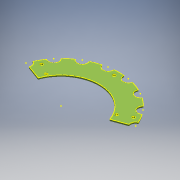
# Autodesk Inventor part: Board_Shape
Saved by Autodesk Inventor 2016 (Build 200138000, 138)
## iProperties
Created: 2015-07-29
Part Number: Board_Shape
Material: Generic
Document SubType Name: Modeling
Designer: bastli
Density: 1 g/cm^3
Appearance: Olive Green
Author: bastli
Autodesk Inventor part; units mm, degrees
ref_plane "YZ Plane" through (0, 0, 0) normal (1, 0, 0) x (0, 1, 0)
ref_plane "XZ Plane" through (0, 0, 0) normal (0, 1, 0) x (-1, 0, 0)
ref_plane "XY Plane" through (0, 0, 0) normal (0, 0, 1) x (1, 0, 0)
sketch "Sketch1" plane through (0, 0, 0) normal (0, 0, 1) x (1, 0, 0)
  arc A0 (65.342, -17.4038) -> (61.2418, -28.669) centre (63.542, -23.1274) ccw projected
  arc A1 (65.342, -17.4038) -> (65.342, 17.4038) centre (0, 0) ccw projected
  arc A2 (61.2418, 28.669) -> (65.342, 17.4038) centre (63.542, 23.1274) ccw projected
  arc A3 (61.2418, 28.669) -> (55.4489, 38.7025) centre (0, 0) ccw projected
  arc A4 (47.7431, 47.8859) -> (55.4489, 38.7025) centre (51.7999, 43.4653) ccw projected
  arc A5 (47.7431, 47.8859) -> (38.8679, 55.3331) centre (0, 0) ccw projected
  arc A6 (28.4859, 61.3272) -> (38.8679, 55.3331) centre (33.81, 58.5606) ccw projected
  arc A7 (28.4859, 61.3272) -> (17.5989, 65.2897) centre (0, 0) ccw projected
  arc A8 (5.7928, 67.3714) -> (17.5989, 65.2897) centre (11.7421, 66.5927) ccw projected
  arc A9 (5.7928, 67.3714) -> (-5.7928, 67.3714) centre (0, 0) ccw projected
  arc A10 (-17.5989, 65.2897) -> (-5.7928, 67.3714) centre (-11.7421, 66.5927) ccw projected
  arc A11 (-17.5989, 65.2897) -> (-28.4859, 61.3272) centre (0, 0) ccw projected
  arc A12 (-38.8679, 55.3331) -> (-28.4859, 61.3272) centre (-33.81, 58.5606) ccw projected
  arc A13 (-38.8679, 55.3331) -> (-47.7431, 47.8859) centre (0, 0) ccw projected
  arc A14 (-55.4489, 38.7025) -> (-47.7431, 47.8859) centre (-51.7999, 43.4653) ccw projected
  arc A15 (-55.4489, 38.7025) -> (-61.2418, 28.669) centre (0, 0) ccw projected
  arc A16 (-65.342, 17.4038) -> (-61.2418, 28.669) centre (-63.542, 23.1274) ccw projected
  arc A17 (-65.342, 17.4038) -> (-65.342, -17.4038) centre (0, 0) ccw projected
  arc A18 (-61.2418, -28.669) -> (-65.342, -17.4038) centre (-63.542, -23.1274) ccw projected
  arc A19 (-61.2418, -28.669) -> (-55.4489, -38.7025) centre (0, 0) ccw projected
  arc A20 (-47.7431, -47.8859) -> (-55.4489, -38.7025) centre (-51.7999, -43.4653) ccw projected
  arc A21 (-47.7431, -47.8859) -> (-38.8679, -55.3331) centre (0, 0) ccw projected
  arc A22 (-28.4859, -61.3272) -> (-38.8679, -55.3331) centre (-33.81, -58.5606) ccw projected
  arc A23 (-28.4859, -61.3272) -> (-17.5989, -65.2897) centre (0, 0) ccw projected
  arc A24 (-5.7928, -67.3714) -> (-17.5989, -65.2897) centre (-11.7421, -66.5927) ccw projected
  arc A25 (-5.7928, -67.3714) -> (5.7928, -67.3714) centre (0, 0) ccw projected
  arc A26 (17.5989, -65.2897) -> (5.7928, -67.3714) centre (11.7421, -66.5927) ccw projected
  arc A27 (17.5989, -65.2897) -> (28.4859, -61.3272) centre (0, 0) ccw projected
  arc A28 (38.8679, -55.3331) -> (28.4859, -61.3272) centre (33.81, -58.5606) ccw projected
  arc A29 (38.8679, -55.3331) -> (47.7431, -47.8859) centre (0, 0) ccw projected
  arc A30 (55.4489, -38.7025) -> (47.7431, -47.8859) centre (51.7999, -43.4653) ccw projected
  arc A31 (55.4489, -38.7025) -> (61.2418, -28.669) centre (0, 0) ccw projected
  circle A32 centre (0, 0) radius 44.3 projected
  circle A33 centre (-62.46, -8) radius 1.2 projected
  circle A34 centre (-46.46, 8) radius 1.2 projected
  circle A35 centre (62.46, -8) radius 1.2 projected
  circle A36 centre (46.46, 8) radius 1.2 projected
  circle A37 centre (62.46, 8) radius 1.2 projected
  circle A38 centre (46.46, -8) radius 1.2 projected
  circle A39 centre (-62.46, 8) radius 1.2 projected
  circle A40 centre (-46.46, -8) radius 1.2 projected
  circle A41 centre (-54.46, 0) radius 7.995 projected
  circle A42 centre (54.46, 0) radius 7.995 projected
  circle A43 centre (53.3645, -30.81) radius 1.55 projected
  circle A44 centre (39.6086, -47.2037) radius 1.55 projected
  circle A45 centre (16.1776, -44.4475) radius 1.55 projected
  circle A46 centre (0, -61.62) radius 1.55 projected
  circle A47 centre (-21.0753, -57.9039) radius 1.55 projected
  circle A48 centre (-30.4039, -36.2339) radius 1.55 projected
  circle A49 centre (-53.3645, -30.81) radius 1.55 projected
  circle A50 centre (53.3645, 30.81) radius 1.55 projected
  circle A51 centre (39.6086, 47.2037) radius 1.55 projected
  circle A52 centre (21.0753, 57.9039) radius 1.55 projected
  circle A53 centre (-40.963, 23.65) radius 1.55 projected
  circle A54 centre (-30.4039, 36.2339) radius 1.55 projected
  circle A55 centre (-16.1776, 44.4475) radius 1.55 projected
  circle A56 centre (0, 47.3) radius 1.55 projected
  circle A57 centre (0, 61.62) radius 1.55 projected
  circle A58 centre (-21.0753, 57.9039) radius 1.55 projected
  circle A59 centre (-39.6086, 47.2037) radius 1.55 projected
  circle A60 centre (-53.3645, 30.81) radius 1.55 projected
  circle A61 centre (16.1776, 44.4475) radius 1.55 projected
  circle A62 centre (30.4039, 36.2339) radius 1.55 projected
  circle A63 centre (40.963, 23.65) radius 1.55 projected
  circle A64 centre (-40.963, -23.65) radius 1.55 projected
  circle A65 centre (-39.6086, -47.2037) radius 1.55 projected
  circle A66 centre (-16.1776, -44.4475) radius 1.55 projected
  circle A67 centre (0, -47.3) radius 1.55 projected
  circle A68 centre (21.0753, -57.9039) radius 1.55 projected
  circle A69 centre (30.4039, -36.2339) radius 1.55 projected
  circle A70 centre (40.963, -23.65) radius 1.55 projected
  line L0 (-57.9039, 21.0753) -> (-41.6284, 15.1515)
  line L1 (41.6284, 15.1515) -> (57.9039, 21.0753)
  point P0 (0, 0)
  constraints: 4 end point, 4 point on circle, 2 line through centre
extrude "Extrusion1" add sketch "Sketch1" along normal blind 1.75 contours L1 A32 L0 A16 A15 A14 A13 A12 A11 A10 A9 A8 A7 A6 A5 A4 A3 A2
sketch "Sketch2" plane through (0, 0, 1.75) normal (0, 0, 1) x (1, 0, 0)
  circle A0 centre (-39.6086, 47.2037) radius 1.55 projected
  circle A1 centre (-30.4039, 36.2339) radius 1.55 projected
  circle A2 centre (-16.1776, 44.4475) radius 1.55 projected
  circle A3 centre (-21.0753, 57.9039) radius 1.55 projected
  circle A4 centre (16.1776, 44.4475) radius 1.55 projected
  circle A5 centre (21.0753, 57.9039) radius 1.55 projected
  circle A6 centre (30.4039, 36.2339) radius 1.55 projected
  circle A7 centre (39.6086, 47.2037) radius 1.55 projected
  circle A8 centre (0, 47.3) radius 1.55 projected
  point P0 (0, 0)
extrude "Extrusion2" add sketch "Sketch2" against normal up to surface (1.75 mm away)
sketch "Sketch3" plane through (0, 0, 1.75) normal (0, 0, 1) x (1, 0, 0)
  circle A0 centre (40.963, 23.65) radius 1.55 projected
  circle A1 centre (-53.3645, 30.81) radius 1.55 projected
  circle A2 centre (0, 61.62) radius 1.55 projected
  circle A3 centre (-40.963, 23.65) radius 1.55 projected
  circle A4 centre (53.3645, 30.81) radius 1.55 projected
  arc A5 (61.2418, 28.669) -> (55.4489, 38.7025) centre (0, 0) ccw projected
  arc A6 (47.7431, 47.8859) -> (55.4489, 38.7025) centre (51.7999, 43.4653) ccw projected
  arc A7 (47.7431, 47.8859) -> (38.8679, 55.3331) centre (0, 0) ccw projected
  arc A8 (28.4859, 61.3272) -> (38.8679, 55.3331) centre (33.81, 58.5606) ccw projected
  arc A9 (28.4859, 61.3272) -> (17.5989, 65.2897) centre (0, 0) ccw projected
  arc A10 (5.7928, 67.3714) -> (17.5989, 65.2897) centre (11.7421, 66.5927) ccw projected
  arc A11 (5.7928, 67.3714) -> (-5.7928, 67.3714) centre (0, 0) ccw projected
  arc A12 (-17.5989, 65.2897) -> (-5.7928, 67.3714) centre (-11.7421, 66.5927) ccw projected
  arc A13 (-17.5989, 65.2897) -> (-28.4859, 61.3272) centre (0, 0) ccw projected
  arc A14 (-38.8679, 55.3331) -> (-28.4859, 61.3272) centre (-33.81, 58.5606) ccw projected
  arc A15 (-38.8679, 55.3331) -> (-47.7431, 47.8859) centre (0, 0) ccw projected
  arc A16 (-55.4489, 38.7025) -> (-47.7431, 47.8859) centre (-51.7999, 43.4653) ccw projected
  arc A17 (-55.4489, 38.7025) -> (-61.2418, 28.669) centre (0, 0) ccw projected
  arc A18 (-57.9039, 21.0753) -> (-61.2418, 28.669) centre (-63.542, 23.1274) ccw projected
  line L0 (-57.9039, 21.0753) -> (-41.6284, 15.1515) projected
  arc A19 (41.6284, 15.1515) -> (-41.6284, 15.1515) centre (0, 0) ccw projected
  line L1 (41.6284, 15.1515) -> (57.9039, 21.0753) projected
  arc A20 (61.2418, 28.669) -> (57.9039, 21.0753) centre (63.542, 23.1274) ccw projected
  point P0 (0, 0)
body "Solid1"
